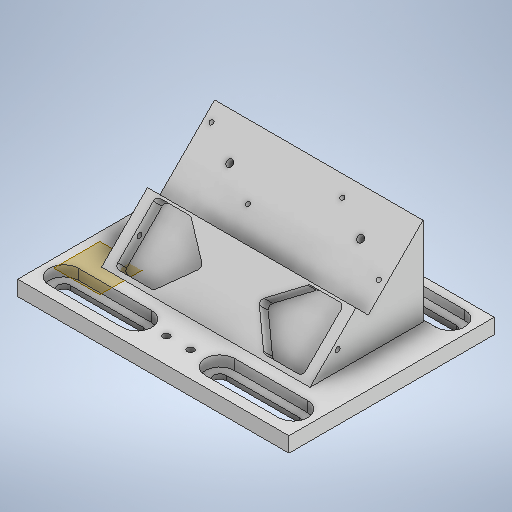
# Autodesk Inventor part: MountCompact1
Saved by Autodesk Inventor 2025 (Build 290162010, 162A)
## iProperties
Created: 2024-12-17
Part Number: MountCompact1
Material: Generic
Document SubType Name: Modeling
Designer: luttmann
Density: 1 g/cm^3
Appearance: Default
Author: luttmann
Autodesk Inventor part; units mm, degrees
note: some values were not read from the file. Chosen so that the rebuilt part matches the saved one: direction of "Hole4"; direction of "Hole5".
ref_plane "YZ Plane" through (0, 0, 0) normal (1, 0, 0) x (0, 1, 0)
ref_plane "XZ Plane" through (0, 0, 0) normal (0, 1, 0) x (-1, 0, 0)
ref_plane "XY Plane" through (0, 0, 0) normal (0, 0, 1) x (1, 0, 0)
sketch "Sketch1" plane through (0, 0, 0) normal (1, 0, 0) x (0, 1, 0)
  line L0 (-1.7454, 18.8803) -> (5.4646, 18.8803)
  line L1 (5.4646, 18.8803) -> (5.4646, -6.1197)
  line L2 (5.4646, -6.1197) -> (65.4646, -66.1197)
  line L3 (65.4646, -66.1197) -> (5.4646, -66.1197)
  line L4 (5.4646, -66.1197) -> (5.4646, -91.1197)
  line L5 (5.4646, -91.1197) -> (-1.7454, -91.1197)
  line L6 (-1.7454, -91.1197) -> (-1.7454, 18.8803)
  point P0 (0, 0)
  dimension "d0" = 25
  dimension "d1" = 25
  dimension "d2" = 7.21
  dimension "d3" = 110
  dimension "d55" = 45
  constraints: 14 end point, 3 perpendicular, 1 horizontal, 1 parallel, 1 point on line
  measures "d0" distance of L0.end L1.end
  measures "d1" distance of L3.end L4.end
  measures "d2" distance of L0.start L0.end
  measures "d3" distance of L5.end L0.start
  measures "d55" angle of L2 L1
extrude "Extrusion1" add sketch "Sketch1" against normal blind 99.5
sketch "Sketch2" plane through (-99.5, 65.4646, -66.1197) normal (0, 0.7071068, 0.7071068) x (1, 0, 0)
  line L0 (94.585, -82.8528) -> (94.585, -54.8528)
  line L1 (94.585, -54.8528) -> (78.085, -54.8528)
  line L2 (78.085, -54.8528) -> (63.085, -67.8528)
  line L3 (63.085, -67.8528) -> (76.085, -82.8528)
  line L4 (76.085, -82.8528) -> (94.585, -82.8528)
  line L5 (99.5, 0) -> (99.5, -84.8528) projected
  line L6 (4.915, -54.8528) -> (4.915, -82.8528)
  line L7 (4.915, -82.8528) -> (23.415, -82.8528)
  line L8 (23.415, -82.8528) -> (36.415, -67.8528)
  line L9 (36.415, -67.8528) -> (21.415, -54.8528)
  line L10 (21.415, -54.8528) -> (4.915, -54.8528)
  line L11 (99.5, -84.8528) -> (0, -84.8528) projected
  line L12 (0, -84.8528) -> (0, 0) projected
  point P0 (99.5, -93.0442)
  dimension "d6" = 28
  dimension "d8" = 31.5
  dimension "d10" = 4.915
  dimension "d11" = 2
  dimension "d12" = 90
  dimension "d13" = 90
  dimension "d14" = 2
  dimension "d16" = 16.5
  dimension "d18" = 31.5
  dimension "d19" = 28
  dimension "d56" = 16.5
  dimension "d57" = 18.5
  dimension "d119" = 4.915
  constraints: 20 end point, 2 parallel, 2 perpendicular, 2 vertical
  measures "d6" distance of L0.start L0.end
  measures "d8" distance from line of L0 L2.end
  measures "d10" distance between parallel lines of L5 L0
  measures "d11" distance between parallel lines of L11 L4
  measures "d12" angle of L2 L3
  measures "d13" angle of L8 L9
  measures "d14" distance between parallel lines of L11 L7
  measures "d16" distance of L9.end L6.start
  measures "d18" distance from line of L6 L8.end
  measures "d19" distance of L6.start L6.end
  measures "d56" distance of L0.end L1.end
  measures "d57" distance of L3.end L0.start
  measures "d119" distance between parallel lines of L12 L6
extrude "Extrusion2" cut sketch "Sketch2" against normal blind 6
sketch "Sketch3" plane through (-99.5, 65.4646, -66.1197) normal (0, 0.7071068, 0.7071068) x (1, 0, 0)
  line L0 (94.585, -54.8528) -> (94.585, -82.8528) projected
  line L1 (4.915, -82.8528) -> (4.915, -54.8528) projected
  line L2 (99.5, 0) -> (99.5, -84.8528) projected
  line L3 (0, -84.8528) -> (0, 0) projected
  point P0 (99.5, -93.0442)
  point P1 (81, -32.8528)
  point P2 (18.5, -32.8528)
  point P3 (94.585, -68.8528)
  point P4 (4.915, -68.8528)
  dimension "d22" = 36
  dimension "d23" = 36
  dimension "d24" = 62.5
  dimension "d25" = 18.5
  dimension "d26" = 18.5
  constraints: 2 midpoint
  measures "d22" vertical distance of point (81, -32.853) point (94.585, -68.853)
  measures "d23" vertical distance of point (18.5, -32.853) point (4.915, -68.853)
  measures "d24" distance of point (81, -32.853) point (18.5, -32.853)
  measures "d25" distance from line of L2 point (81, -32.853)
  measures "d26" distance from line of L3 point (18.5, -32.853)
hole "Hole1" at (-18.5, 42.2342, -42.8892) at (-81, 42.2342, -42.8892) direction (0, -0.7071068, -0.7071068) diameter 3.242 depth 15 tip angle 118 thread size "M4x0.7" class "6H" standard "ANSI Metric M Profile"
sketch "Sketch4" plane through (-99.5, 65.4646, -66.1197) normal (0, 0.7071068, 0.7071068) x (1, 0, 0)
  line L0 (0, -84.8528) -> (0, 0) projected
  line L1 (99.5, 0) -> (0, 0) projected
  line L2 (0, -53.8528) -> (99.5, -53.8528)
  line L3 (99.5, -53.8528) -> (99.5, 0)
  line L4 (99.5, 0) -> (0, 0)
  line L5 (0, 0) -> (0, -53.8528)
  circle A0 centre (81, -32.8528) radius 1.621 projected
  point P0 (99.5, -93.0442)
  dimension "d34" = 21
  constraints: 8 end point, 2 parallel, 1 horizontal, 1 perpendicular, 1 point on line
  measures "d34" distance from line of L2 A0.centre
extrude "Extrusion3" cut sketch "Sketch4" against normal blind 8.4
sketch "Sketch10" plane through (0, 0, 0) normal (1, 0, 0) x (0, 0, -1)
  line L0 (91.1197, 5.4646) -> (66.1197, 5.4646) projected
  line L1 (66.1197, 5.4646) -> (60.1197, 5.4646)
  line L2 (60.1197, 5.4646) -> (60.1197, 47.5852)
  line L3 (33.9797, 21.4452) -> (66.1197, 53.5852) projected
  line L4 (60.1197, 47.5852) -> (66.1197, 53.5852)
  line L5 (66.1197, 53.5852) -> (66.1197, 5.4646)
  point P0 (0, 0)
  dimension "d58" = 6
  constraints: 8 end point, 2 perpendicular, 1 collinear, 1 horizontal, 1 point on line
  measures "d58" distance of L0.end L1.end
extrude "Extrusion8" cut sketch "Sketch10" against normal through all
sketch "Sketch11" plane through (-99.5, 59.5249, -72.0594) normal (0, 0.7071068, 0.7071068) x (1, 0, 0)
  circle A0 centre (81, -32.8528) radius 1.621 projected
  circle A1 centre (18.5, -32.8528) radius 1.621 projected
  point P0 (99.5, -93.0442)
  point P1 (66, -23.9528)
  point P2 (96, -41.7528)
  point P3 (3.5, -23.9528)
  point P4 (33.5, -41.7528)
  dimension "d61" = 15
  dimension "d62" = 15
  dimension "d63" = 8.9
  dimension "d64" = 8.9
  dimension "d65" = 8.9
  dimension "d66" = 8.9
  dimension "d67" = 15
  dimension "d68" = 15
  measures "d61" horizontal distance of point (96, -41.753) A0.centre
  measures "d62" horizontal distance of A0.centre point (66, -23.953)
  measures "d63" vertical distance of A0.centre point (66, -23.953)
  measures "d64" vertical distance of point (96, -41.753) A0.centre
  measures "d65" vertical distance of A1.centre point (3.5, -23.953)
  measures "d66" vertical distance of A1.centre point (33.5, -41.753)
  measures "d67" horizontal distance of A1.centre point (3.5, -23.953)
  measures "d68" horizontal distance of A1.centre point (33.5, -41.753)
hole "Hole2" at (-33.5, 42.5877, -55.1222) at (-3.5, 30.0012, -42.5357) at (-96, 42.5877, -55.1222) at (-66, 30.0012, -42.5357) direction (0, -0.7071068, -0.7071068) diameter 2 depth 4 tip angle 118
sketch "Sketch12" plane through (-99.5, 5.4646, -91.1197) normal (0, 1, 0) x (1, 0, 0)
  arc A0 (36, -101) -> (36, -95) centre (36, -98) ccw projected
  arc A1 (1, -95) -> (1, -101) centre (1, -98) ccw projected
  line L0 (99.5, 0) -> (99.5, -31) projected
  line L1 (0, -31) -> (0, 0) projected
  point P0 (99.5, -91.1197)
  point P1 (18.5, -23)
  point P2 (0, -15.5)
  dimension "d79" = 75
  dimension "d120" = 18.5
  constraints: 1 midpoint
  measures "d79" vertical distance of A1.centre point (18.5, -23)
  measures "d120" distance from line of L1 point (18.5, -23)
hole "Hole3" at (-81, 5.4646, -68.1197) direction (0, -1, 0) diameter 6 end through all counterbore diameter 14.55 counterbore depth 4.38 clearance for "Hex Head Bolt" size "M6" standard "Ansi Metric M Profile"
sketch "Sketch14" plane through (0, 0, 0) normal (1, 0, 0) x (0, 0, -1)
  line L0 (60.1197, 5.4646) -> (91.1197, 5.4646) projected
  line L1 (91.1197, -1.7454) -> (-18.8803, -1.7454) projected
  line L2 (91.1197, 5.4646) -> (79.1197, 5.4646)
  line L3 (79.1197, 5.4646) -> (79.1197, -1.7454)
  line L4 (79.1197, -1.7454) -> (91.1197, -1.7454)
  line L5 (91.1197, -1.7454) -> (91.1197, 5.4646)
  point P0 (0, 0)
  dimension "d95" = 12
  constraints: 8 end point, 2 parallel, 1 horizontal, 1 perpendicular, 1 point on line
  measures "d95" distance between parallel lines of L5 L3
extrude "Extrusion10" cut sketch "Sketch14" against normal through all
fillet "Fillet1" radius 2 10 edges at (-94.585, 4.7568, -9.6559) (-94.585, 24.5558, -29.4549) (-78.085, 24.5558, -29.4549) (-63.085, 15.3634, -20.2625) (-76.085, 4.7568, -9.6559) (-4.915, 4.7568, -9.6559) (-21.415, 24.5558, -29.4549) (-4.915, 24.5558, -29.4549) (-23.415, 4.7568, -9.6559) (-36.415, 15.3634, -20.2625)
sketch "Sketch15" plane through (0, 0, 0) normal (1, 0, 0) x (0, 0, -1)
  line L0 (28.04, 27.3849) -> (6.1197, 5.4646) projected
  line L1 (33.9797, 21.4452) -> (28.04, 27.3849) projected
  point P0 (0, 0)
  point P1 (19.3426, 14.4449)
  point P2 (6.7055, 6.0504)
  point P3 (32.5655, 22.8595)
  dimension "d101" = 3
  dimension "d102" = 15.3
  measures "d101" distance from line of L0 point (19.343, 14.445)
  measures "d102" distance from line of L1 point (19.343, 14.445)
hole "Hole4" at (0, 14.4449, -19.3426) direction (-1, 0, 0) diameter 2.459 depth 4.915 thread size "M3x0.5" class "6H" standard "ANSI Metric M Profile"
sketch "Sketch16" plane through (-99.5, 0, 0) normal (-1, 0, 0) x (0, 0, 1)
  circle A0 centre (-19.3426, 14.4449) radius 1.2295 projected
  line L0 (-6.1197, 5.4646) -> (-28.04, 27.3849) projected
  line L1 (-28.04, 27.3849) -> (-33.9797, 21.4452) projected
  point P0 (0, 0)
  point P1 (-6.7055, 6.0504)
  point P2 (-32.5655, 22.8595)
  dimension "d110" = 3
  dimension "d111" = 15.3
  constraints: 1 coincident
  measures "d110" distance from line of L0 A0.centre
  measures "d111" distance from line of L1 A0.centre
hole "Hole5" at (-99.5, 14.4449, -19.3426) direction (1, 0, 0) diameter 2.459 depth 4.915 thread size "M3x0.5" class "6H" standard "ANSI Metric M Profile"
sketch "Sketch17" plane through (-99.5, 5.4646, -60.1197) normal (0, 1, 0) x (1, 0, 0)
  line L0 (99.5, -79) -> (99.5, 19) projected
  line L1 (99.5, 19) -> (114.5, 19)
  line L2 (114.5, 19) -> (114.5, 0)
  line L3 (114.5, 0) -> (99.5, 0)
  line L4 (99.5, 0) -> (99.5, 19)
  line L5 (0, 19) -> (0, -79) projected
  line L6 (0, 19) -> (-15, 19)
  line L7 (-15, 19) -> (-15, 0)
  line L8 (-15, 0) -> (0, 0)
  line L9 (0, 0) -> (0, 19)
  line L10 (99.5, -79) -> (114.5, -79)
  line L11 (114.5, -79) -> (114.5, -54.8353)
  line L12 (114.5, -54.8353) -> (99.5, -54.8353)
  line L13 (99.5, -54.8353) -> (99.5, -79)
  line L14 (0, -79) -> (-15, -79)
  line L15 (-15, -79) -> (-15, -54.8353)
  line L16 (-15, -54.8353) -> (0, -54.8353)
  line L17 (0, -54.8353) -> (0, -79)
  point P0 (99.5, -60.1197)
  dimension "d121" = 19
  dimension "d122" = 15
  dimension "d123" = 15
  dimension "d124" = 24.1647
  dimension "d125" = 24.1647
  dimension "d126" = 15
  dimension "d127" = 19
  dimension "d128" = 15
  constraints: 32 end point, 8 parallel, 4 horizontal, 4 perpendicular, 3 point on line
  measures "d121" distance of L1.end L2.end
  measures "d122" distance of L0.end L1.end
  measures "d123" distance of L10.start L10.end
  measures "d124" distance of L10.end L11.end
  measures "d125" distance of L14.end L15.end
  measures "d126" distance of L5.end L14.end
  measures "d127" distance of L6.end L7.end
  measures "d128" distance of L5.start L6.end
extrude "Extrusion11" add sketch "Sketch17" against normal blind 7.21
sketch "Sketch18" plane through (-114.5, 5.4646, -60.1197) normal (0, 1, 0) x (1, 0, 0)
  line L0 (51.5, 8) -> (119.5, 8) construction
  line L1 (51.5, 1) -> (119.5, 1)
  line L2 (119.5, 15) -> (51.5, 15)
  arc A0 (51.5, 15) -> (51.5, 1) centre (51.5, 8) ccw
  arc A1 (119.5, 1) -> (119.5, 15) centre (119.5, 8) ccw
  line L3 (9, 8) -> (16, 8) construction
  line L4 (9, 15) -> (16, 15)
  line L5 (16, 1) -> (9, 1)
  arc A2 (9, 15) -> (9, 1) centre (9, 8) ccw
  arc A3 (16, 1) -> (16, 15) centre (16, 8) ccw
  line L6 (0, 19) -> (0, 0) projected
  line L7 (129.5, 0) -> (129.5, 19) projected
  line L8 (0, 0) -> (15, 0) projected
  arc A4 (16, -60) -> (16, -74) centre (16, -67) ccw projected
  arc A5 (51, -74) -> (51, -60) centre (51, -67) ccw projected
  point P0 (114.5, -60.1197)
  point P1 (85.5, 8)
  point P2 (12.5, 8)
  dimension "d131" = 7
  dimension "d132" = 7
  dimension "d133" = 9
  dimension "d134" = 7
  dimension "d135" = 10
  dimension "d136" = 68
  dimension "d138" = 75
  dimension "d139" = 75
  constraints: 16 end point, 8 point on circle, 8 tangent, 4 centre point, 2 midpoint, 2 parallel, 2 point on line, 1 horizontal
  measures "d131" radius of A0
  measures "d132" radius of A2
  measures "d133" distance from line of L6 L3.start
  measures "d134" distance of L3.start L3.end
  measures "d135" distance from line of L7 L0.end
  measures "d136" distance of L0.start L0.end
  measures "d138" vertical distance of A4.centre L3.start
  measures "d139" vertical distance of A5.centre L0.end
extrude "Extrusion12" cut sketch "Sketch18" against normal blind 4.38
sketch "Sketch19" plane through (-114.5, 1.0846, -60.1197) normal (0, 1, 0) x (1, 0, 0)
  arc A0 (9, 15) -> (9, 1) centre (9, 8) ccw projected
  arc A1 (16, 1) -> (16, 15) centre (16, 8) ccw projected
  line L0 (9, 8) -> (16, 8) construction
  line L1 (9, 5) -> (16, 5)
  line L2 (16, 11) -> (9, 11)
  arc A2 (9, 11) -> (9, 5) centre (9, 8) ccw
  arc A3 (16, 5) -> (16, 11) centre (16, 8) ccw
  arc A4 (51.5, 15) -> (51.5, 1) centre (51.5, 8) ccw projected
  arc A5 (119.5, 1) -> (119.5, 15) centre (119.5, 8) ccw projected
  line L3 (51.5, 8) -> (119.5, 8) construction
  line L4 (51.5, 5) -> (119.5, 5)
  line L5 (119.5, 11) -> (51.5, 11)
  arc A6 (51.5, 11) -> (51.5, 5) centre (51.5, 8) ccw
  arc A7 (119.5, 5) -> (119.5, 11) centre (119.5, 8) ccw
  point P0 (114.5, -60.1197)
  point P1 (12.5, 8)
  point P2 (85.5, 8)
  dimension "d142" = 3
  dimension "d143" = 3
  constraints: 16 end point, 8 point on circle, 8 tangent, 4 centre point, 3 parallel, 2 midpoint, 1 horizontal
  measures "d142" radius of A2
  measures "d143" radius of A6
extrude "Extrusion13" cut sketch "Sketch19" against normal through all
ref_plane "Work Plane2" through (-99.5, 5.4646, -5.2913) normal (0, 1, 0) x (1, 0, 0)
sketch "Sketch20" plane through (-99.5, 5.4646, -5.2913) normal (0, 1, 0) x (1, 0, 0)
  line L0 (-5, -12.1716) -> (30, -12.1716) construction
  line L1 (-5, -19.1716) -> (30, -19.1716)
  line L2 (30, -5.1716) -> (-5, -5.1716)
  arc A0 (-5, -5.1716) -> (-5, -19.1716) centre (-5, -12.1716) ccw
  arc A1 (30, -19.1716) -> (30, -5.1716) centre (30, -12.1716) ccw
  line L3 (69.5, -12.1716) -> (104.5, -12.1716) construction
  line L4 (69.5, -19.1716) -> (104.5, -19.1716)
  line L5 (104.5, -5.1716) -> (69.5, -5.1716)
  arc A2 (69.5, -5.1716) -> (69.5, -19.1716) centre (69.5, -12.1716) ccw
  arc A3 (104.5, -19.1716) -> (104.5, -5.1716) centre (104.5, -12.1716) ccw
  circle A4 centre (18.5, 62.8284) radius 3 projected
  circle A5 centre (18.5, 62.8284) radius 7.275 projected
  line L6 (-15, -0.0069) -> (-15, -24.1716) projected
  line L7 (114.5, -24.1716) -> (114.5, -0.0069) projected
  point P0 (99.5, -5.2913)
  point P1 (12.5, -12.1716)
  point P2 (87, -12.1716)
  dimension "d153" = 75
  dimension "d154" = 75
  dimension "d155" = 10
  dimension "d156" = 10
  dimension "d157" = 7
  dimension "d158" = 7
  dimension "d159" = 35
  dimension "d160" = 35
  constraints: 16 end point, 8 point on circle, 8 tangent, 4 centre point, 2 midpoint, 2 parallel, 2 point on line, 1 horizontal
  measures "d153" distance from line of A4.centre L0
  measures "d154" vertical distance of A5.centre L3.end
  measures "d155" distance from line of L6 L0.start
  measures "d156" distance from line of L7 L3.end
  measures "d157" radius of A0
  measures "d158" radius of A3
  measures "d159" distance of L1.start L1.end
  measures "d160" distance of L4.start L4.end
extrude "Extrusion14" cut sketch "Sketch20" against normal blind 5 contours A0 L2 A1 L1 | A2 L5 A3 L4
sketch "Sketch21" plane through (-99.5, 0.4646, -5.2913) normal (0, 1, 0) x (1, 0, 0)
  arc A0 (-5, -5.1716) -> (-5, -19.1716) centre (-5, -12.1716) ccw projected
  arc A1 (30, -19.1716) -> (30, -5.1716) centre (30, -12.1716) ccw projected
  line L0 (-5, -12.1716) -> (30, -12.1716) construction
  line L1 (-5, -15.1716) -> (30, -15.1716)
  line L2 (30, -9.1716) -> (-5, -9.1716)
  arc A2 (-5, -9.1716) -> (-5, -15.1716) centre (-5, -12.1716) ccw
  arc A3 (30, -15.1716) -> (30, -9.1716) centre (30, -12.1716) ccw
  arc A4 (69.5, -5.1716) -> (69.5, -19.1716) centre (69.5, -12.1716) ccw projected
  arc A5 (104.5, -19.1716) -> (104.5, -5.1716) centre (104.5, -12.1716) ccw projected
  line L3 (69.5, -12.1716) -> (104.5, -12.1716) construction
  line L4 (69.5, -15.1716) -> (104.5, -15.1716)
  line L5 (104.5, -9.1716) -> (69.5, -9.1716)
  arc A6 (69.5, -9.1716) -> (69.5, -15.1716) centre (69.5, -12.1716) ccw
  arc A7 (104.5, -15.1716) -> (104.5, -9.1716) centre (104.5, -12.1716) ccw
  point P0 (99.5, -5.2913)
  point P1 (12.5, -12.1716)
  point P2 (87, -12.1716)
  dimension "d163" = 3
  dimension "d164" = 3
  constraints: 16 end point, 8 point on circle, 8 tangent, 4 centre point, 2 horizontal, 2 midpoint, 2 parallel
  measures "d163" radius of A2
  measures "d164" radius of A7
extrude "Extrusion15" cut sketch "Sketch21" against normal through all
ref_plane "Work Plane1" through (-99.5, 5.4646, -5.2913) normal (0, 1, 0) x (1, 0, 0)
sketch "Sketch22" plane through (-99.5, 5.4646, -5.2913) normal (0, 1, 0) x (1, 0, 0)
  line L0 (-15, -24.1716) -> (114.5, -24.1716)
  line L1 (114.5, -24.1716) -> (114.5, -0.0069) projected
  line L2 (-15, -0.0069) -> (-15, -24.1716) projected
  point P0 (99.5, -5.2913)
  point P1 (44, -12.1716)
  point P2 (55.5, -12.1716)
  dimension "d167" = 12
  dimension "d168" = 12
  dimension "d169" = 59
  dimension "d170" = 59
  constraints: 2 end point
  measures "d167" distance from line of L0 point (44, -12.172)
  measures "d168" distance from line of L0 point (55.5, -12.172)
  measures "d169" distance from line of L1 point (55.5, -12.172)
  measures "d170" distance from line of L2 point (44, -12.172)
hole "Hole6" at (-55.5, 5.4646, 6.8803) at (-44, 5.4646, 6.8803) direction (0, -1, 0) diameter 3.242 end through all thread size "M4x0.7" class "6H" standard "ANSI Metric M Profile"
sketch "Sketch23" plane through (0, 0, 0) normal (1, 0, 0) x (0, 0, -1)
  line L0 (5.2843, -1.7454) -> (60.1197, -1.7454) projected
  line L1 (5.2843, 5.4646) -> (60.1197, 5.4646)
  line L2 (60.1197, 5.4646) -> (60.1197, -1.7454)
  line L3 (60.1197, -1.7454) -> (5.2843, -1.7454)
  line L4 (5.2843, -1.7454) -> (5.2843, 5.4646)
  point P0 (0, 0)
  dimension "d178" = 7.21
  dimension "d179" = 54.8353
  constraints: 8 end point, 2 parallel, 1 horizontal, 1 perpendicular
  measures "d178" distance of L3.end L1.start
  measures "d179" distance of L0.start L0.end
extrude "Extrusion16" add sketch "Sketch23" along normal blind 15
sketch "Sketch24" plane through (-99.5, 0, 0) normal (-1, 0, 0) x (0, 0, 1)
  line L0 (-60.1197, 47.5852) -> (-60.1197, 5.4646) projected
  line L1 (-60.1197, -1.7454) -> (-5.2843, -1.7454) projected
  line L2 (-60.1197, 5.4646) -> (-5.2843, 5.4646)
  line L3 (-5.2843, 5.4646) -> (-5.2843, -1.7454)
  line L4 (-5.2843, -1.7454) -> (-60.1197, -1.7454)
  line L5 (-60.1197, -1.7454) -> (-60.1197, 5.4646)
  point P0 (0, 0)
  dimension "d182" = 7.21
  dimension "d183" = 54.8353
  constraints: 8 end point, 2 parallel, 1 horizontal, 1 perpendicular
  measures "d182" distance of L4.end L0.end
  measures "d183" distance of L1.start L1.end
extrude "Extrusion17" add sketch "Sketch24" along normal blind 15
equation "\"d16\" = d7"
equation "\"d23\" = d22"
equation "\"d7\" = 16.5"
body "Solid1"
